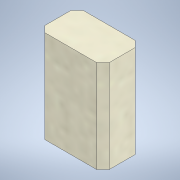
# Autodesk Inventor part: ControlMarker_All
Saved by Autodesk Inventor 2021 (Build 250183000, 183)
## iProperties
Created: 2023-03-16
Part Number: ControlMarker_All
Material: Paper
Document SubType Name: Modeling
Designer: Bradley
Density: 0.93 g/cm^3
Appearance: Cardboard - Chipboard
CMLength: 12.500 mm
CMWidth: 20.900 mm
CMChamfer: 2.000 mm
Author: Bradley
Autodesk Inventor part; units mm, degrees
ref_plane "YZ Plane" through (0, 0, 0) normal (1, 0, 0) x (0, 1, 0)
ref_plane "XZ Plane" through (0, 0, 0) normal (0, 1, 0) x (-1, 0, 0)
ref_plane "XY Plane" through (0, 0, 0) normal (0, 0, 1) x (1, 0, 0)
sketch "Sketch1" plane through (0, 0, 0) normal (0, 1, 0) x (-1, 0, 0)
  line L0 (8.45, 6.25) -> (-8.45, 6.25)
  line L1 (-10.45, 4.25) -> (-10.45, -4.25)
  line L2 (-8.45, -6.25) -> (8.45, -6.25)
  line L3 (10.45, -4.25) -> (10.45, 4.25)
  line L4 (10.45, 6.25) -> (-10.45, -6.25) construction
  line L5 (-10.45, 6.25) -> (10.45, -6.25) construction
  line L6 (8.45, -6.25) -> (10.45, -4.25)
  line L7 (10.45, 4.25) -> (8.45, 6.25)
  line L8 (-8.45, 6.25) -> (-10.45, 4.25)
  line L9 (-10.45, -4.25) -> (-8.45, -6.25)
  point P0 (0, 0)
  dimension "d0" = 20.9
  dimension "d1" = 12.5
  dimension "d2" = 2
  dimension "d3" = 2
  constraints: 20 end point, 8 point on line, 7 perpendicular, 2 midpoint, 2 parallel, 1 horizontal
  measures "d0" distance of L5.end L4.end
  measures "d1" distance of L4.end L5.start
  measures "d2" distance of L2.end L5.end
  measures "d3" distance of L3.start L5.end
extrude "Extrusion1" add sketch "Sketch1" along normal mid plane 30.1
equation "\"d0\" = CMWidth"
equation "\"d1\" = CMLength"
equation "\"d2\" = CMChamfer"
equation "\"d3\" = d2"
equation "\"CMWidth\" = 20.9"
equation "\"CMLength\" = 12.5"
equation "\"CMChamfer\" = 2"
body "Solid1"
